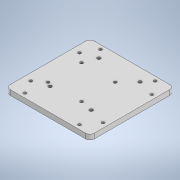
# Autodesk Inventor part: EboxMounting_Plate
Saved by Autodesk Inventor 2022 (Build 260153000, 153)
## iProperties
Created: 2021-10-09
Part Number: EboxMounting_Plate
Material: Generic
Document SubType Name: Modeling
Designer: Jorian Brusind
Density: 1 g/cm^3
Appearance: Default
Author: Jorian Brusind
Autodesk Inventor part; units mm, degrees
ref_plane "YZ Plane" through (0, 0, 0) normal (1, 0, 0) x (0, 1, 0)
ref_plane "XZ Plane" through (0, 0, 0) normal (0, 1, 0) x (-1, 0, 0)
ref_plane "XY Plane" through (0, 0, 0) normal (0, 0, 1) x (1, 0, 0)
sketch "Sketch2" plane through (0, 0, 0) normal (0, 1, 0) x (-1, 0, 0)
  line L0 (0, 0) -> (100, 0)
  line L1 (100, 0) -> (100, -100)
  line L2 (100, -100) -> (0, -100)
  line L3 (0, -100) -> (0, 0)
  circle A0 centre (82.5, -5) radius 1.75
  circle A1 centre (82.5, -95) radius 1.75
  circle A2 centre (17.5, -5) radius 1.75
  circle A3 centre (17.5, -95) radius 1.75
  circle A4 centre (80, -30) radius 1.75
  circle A5 centre (91.5, -21) radius 1.75
  circle A6 centre (91.5, -79) radius 1.75
  circle A7 centre (5.5, -21) radius 1.75
  circle A8 centre (5.5, -79) radius 1.75
  line L4 (50, 0) -> (50, -100)
  circle A9 centre (40, -30) radius 1.75
  circle A10 centre (80, -70) radius 1.75
  circle A11 centre (40, -70) radius 1.75
  dimension "d13" = 100
  dimension "d14" = 100
  dimension "d15" = 3.5
  dimension "d16" = 17.5
  dimension "d17" = 5
  dimension "d20" = 90
  dimension "d23" = 65
  dimension "d26" = 3.5
  dimension "d27" = 20
  dimension "d28" = 30
  dimension "d32" = 3.5
  dimension "d35" = 58
  dimension "d38" = 86
  dimension "d41" = 8.5
  dimension "d42" = 21
  dimension "d51" = 40
  dimension "d54" = 40
  constraints: 12 centre point, 10 end point, 4 horizontal, 3 vertical, 2 midpoint, 2 parallel, 1 perpendicular, 18 other
  measures "d13" distance of L1.end L2.end
  measures "d14" distance of L0.end L1.end
  measures "d15" diameter of A0
  measures "d16" distance from line of L1 A0.centre
  measures "d17" distance from line of L0 A0.centre
  measures "d20" distance of A0.centre A1.centre
  measures "d23" distance of A0.centre A2.centre
  measures "d26" diameter of A4
  measures "d27" distance from line of L1 A4.centre
  measures "d28" distance from line of L0 A4.centre
  measures "d32" diameter of A5
  measures "d35" distance of A5.centre A6.centre
  measures "d38" distance of A5.centre A7.centre
  measures "d41" distance from line of L1 A5.centre
  measures "d42" distance from line of L0 A5.centre
  measures "d51" distance of A4.centre A9.centre
  measures "d54" distance of A4.centre A10.centre
extrude "Extrusion2" add sketch "Sketch2" along normal blind 6
fillet "Fillet2" radius 5 4 edges at (0, 3, -100) (-100, 3, -100) (0, 3, 0) (-100, 3, 0)
sketch "Sketch3" plane through (0, 6, 0) normal (0, 1, 0) x (1, 0, 0)
  circle A0 centre (-74.5, 27) radius 2
  line L0 (-100, 95) -> (-100, 5) projected
  line L1 (-95, 0) -> (-5, 0) projected
  circle A1 centre (-25.5, 27) radius 2
  circle A2 centre (-74.5, 85) radius 2
  circle A3 centre (-25.5, 85) radius 2
  point P0 (0, 0)
  dimension "d57" = 4
  dimension "d58" = 25.5
  dimension "d59" = 27
  dimension "d62" = 49
  dimension "d65" = 58
  constraints: 4 centre point, 1 horizontal, 1 vertical, 6 other
  measures "d57" diameter of A0
  measures "d58" distance from line of L0 A0.centre
  measures "d59" distance from line of L1 A0.centre
  measures "d62" distance of A0.centre A1.centre
  measures "d65" distance of A0.centre A2.centre
extrude "Extrusion3" cut sketch "Sketch3" against normal through all
body "Solid2"
